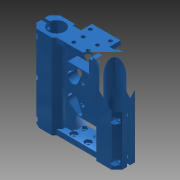
# Autodesk Inventor part: ChimeraXCarriage4
Saved by Autodesk Inventor 2015 SP1 (Build 190203100, 203)
## iProperties
Created: 2015-01-02
Part Number: ChimeraXCarriage4
Material: ABS Plastic
Document SubType Name: Modeling
Designer: Jack
Density: 1.06 g/cm^3
Appearance: Cyan
Mass: 64.3175 g
Surface Area: 300.836 cm^2
Volume: 60.6769 cm^3
Author: Jack
Autodesk Inventor part; units mm, degrees
ref_plane "YZ Plane" through (0, 0, 0) normal (1, 0, 0) x (0, 1, 0)
ref_plane "XZ Plane" through (0, 0, 0) normal (0, 1, 0) x (-1, 0, 0)
ref_plane "XY Plane" through (0, 0, 0) normal (0, 0, 1) x (1, 0, 0)
sketch "Sketch1" plane through (0, 0, 0) normal (0, 0, 1) x (1, 0, 0)
  arc A0 (-7.6035, -1.5) -> (-7.6035, 1.5) centre (0, 0) ccw
  arc A1 (62.6035, 1.5) -> (62.6035, -1.5) centre (55, 0) ccw
  line L0 (-7.6035, 1.5) -> (-13, 1.5)
  line L1 (-13, 1.5) -> (-13, 11)
  line L2 (-13, 11) -> (11.5, 11)
  line L3 (11.5, 11) -> (11.5, 6)
  line L4 (11.5, 6) -> (43.5, 6)
  line L5 (43.5, 6) -> (43.5, 11)
  line L6 (43.5, 11) -> (68, 11)
  line L7 (68, 11) -> (68, 1.5)
  line L8 (68, 1.5) -> (62.6035, 1.5)
  line L9 (62.6035, -1.5) -> (68, -1.5)
  line L10 (68, -1.5) -> (68, -11)
  line L11 (-13, -11) -> (-13, -1.5)
  line L12 (-13, -1.5) -> (-7.6035, -1.5)
  line L13 (-13, -11) -> (11.5, -11)
  line L14 (11.5, -11) -> (11.5, -3)
  line L15 (11.5, -3) -> (43.5, -3)
  line L16 (43.5, -3) -> (43.5, -11)
  line L17 (43.5, -11) -> (68, -11)
  dimension "d0" = 15.5
  dimension "d1" = 15.5
  dimension "d2" = 55
  dimension "d3" = 1.5
  dimension "d4" = 13
  dimension "d5" = 11
  dimension "d6" = 11
  dimension "d7" = 11.5
  dimension "d8" = 11.5
  dimension "d9" = 5
  dimension "d10" = 8
  constraints: 36 end point, 11 perpendicular, 7 point on line, 4 horizontal alignment, 4 point on circle, 3 equal length, 3 horizontal, 2 centre point, 2 vertical alignment, 1 coincident, 1 parallel
  measures "d0" diameter of A0
  measures "d1" diameter of A1
  measures "d2" distance of point (0, 0) A1.centre
  measures "d3" distance from line of point (0, 0) L0
  measures "d4" distance from line of point (0, 0) L1
  measures "d5" distance from line of L2 point (0, 0)
  measures "d6" distance from line of L13 point (0, 0)
  measures "d7" distance from line of L3 point (0, 0)
  measures "d8" distance from line of L5 A1.centre
  measures "d9" distance of L2.end L3.end
  measures "d10" distance of L13.end L14.end
extrude "Extrusion1" add sketch "Sketch1" along normal blind 80
chamfer "Chamfer1" distance 5 angle 45 4 edges at (-13, 11, 40) (-13, -11, 40) (68, 11, 40) (68, -11, 40)
chamfer "Chamfer2" distance 5 angle 45 2 edges at (11.5, 11, 40) (43.5, 11, 40)
chamfer "Chamfer3" distance 5 angle 45 2 edges at (11.5, -11, 40) (43.5, -11, 40)
sketch "Sketch2" plane through (0, 0, 80) normal (0, 0, 1) x (1, 0, 0)
  line L0 (48.5, -11) -> (43.5, -6) projected
  line L1 (48.5, -11) -> (63, -11) projected
  line L2 (63, 11) -> (48.5, 11) projected
  line L3 (43.5, 6) -> (48.5, 11) projected
  line L4 (43.5, 6) -> (11.5, 6) projected
  line L5 (6.5, 11) -> (11.5, 6) projected
  line L6 (11.5, -6) -> (11.5, -3) projected
  line L7 (11.5, -3) -> (43.5, -3) projected
  line L8 (43.5, -3) -> (43.5, -6) projected
  line L9 (8.8, 8.7) -> (46.2, 8.7)
  line L10 (6.5, -11) -> (11.5, -6) projected
  line L11 (8.8, -8.7) -> (46.2, -8.7)
  dimension "d22" = 2.3
  dimension "d23" = 2.3
  constraints: 4 end point, 4 point on line, 1 horizontal, 1 parallel
  measures "d22" distance between parallel lines of L1 L11
  measures "d23" distance between parallel lines of L2 L9
extrude "Extrusion2" add sketch "Sketch2" against normal blind 5
sketch "Sketch3" plane through (0, 0, 0) normal (0, 0, -1) x (-1, 0, 0)
  line L0 (-43.5, -6) -> (-48.5, -11) projected
  line L1 (-43.5, -3) -> (-43.5, -6) projected
  line L2 (-11.5, -3) -> (-43.5, -3) projected
  line L3 (-11.5, -6) -> (-11.5, -3) projected
  line L4 (-6.5, -11) -> (-11.5, -6) projected
  line L5 (-11.5, 6) -> (-6.5, 11) projected
  line L6 (-43.5, 6) -> (-11.5, 6) projected
  line L7 (-48.5, 11) -> (-43.5, 6) projected
  line L8 (-8.8, 8.7) -> (-46.2, 8.7) projected
  line L9 (-46.2, -8.7) -> (-8.8, -8.7) projected
extrude "Extrusion3" add sketch "Sketch3" against normal blind 5
sketch "Sketch4" plane through (11.5, 6, 75) normal (0, 1, 0) x (1, 0, 0)
  line L0 (0, 0) -> (32, 0) projected
  line L1 (0, 70) -> (32, 70) projected
  line L2 (30, 70) -> (10, 70)
  line L3 (10, 70) -> (10, 55)
  line L4 (10, 55) -> (30, 55)
  line L5 (30, 55) -> (30, 70)
  line L6 (22, 0) -> (2, 0)
  line L7 (2, 0) -> (2, 15)
  line L8 (2, 15) -> (22, 15)
  line L9 (22, 15) -> (22, 0)
  line L10 (0, 70) -> (0, 0) projected
  line L11 (32, 70) -> (32, 0) projected
  point P0 (-11.5, 75)
  dimension "d28" = 20
  dimension "d29" = 15
  dimension "d33" = 2
  dimension "d34" = 2
  constraints: 16 end point, 6 parallel, 2 horizontal, 2 perpendicular, 2 point on line
  measures "d28" distance of L4.end L3.end
  measures "d29" distance of L3.end L2.end
  measures "d33" distance between parallel lines of L10 L7
  measures "d34" distance between parallel lines of L11 L5
extrude "Extrusion4" cut sketch "Sketch4" against normal up to next contours L7 L8 L9 L0 | L1 L5 L4 L3
sketch "Sketch5" plane through (43.5, 6, 75) normal (0, 1, 0) x (1, 0, 0)
  line L0 (-10, 0) -> (0, 0) projected
  line L1 (0, 70) -> (0, 0) projected
  circle A0 centre (-16, 44) radius 1.75
  circle A1 centre (-16, 26) radius 1.75
  point P0 (-43.5, 75)
  dimension "d35" = 3.5
  dimension "d36" = 3.5
  dimension "d37" = 16
  dimension "d38" = 18
  dimension "d39" = 26
  constraints: 2 centre point, 1 vertical alignment
  measures "d35" diameter of A0
  measures "d36" diameter of A1
  measures "d37" distance from line of L1 A1.centre
  measures "d38" distance of A0.centre A1.centre
  measures "d39" distance from line of L0 A1.centre
extrude "Extrusion5" cut sketch "Sketch5" against normal up to next
sketch "Sketch6" plane through (43.5, 6, 75) normal (0, 1, 0) x (1, 0, 0)
  circle A0 centre (-16, 44) radius 1.75 projected
  circle A1 centre (-16, 26) radius 1.75 projected
  circle A2 centre (-25, 44) radius 5
  circle A3 centre (-25, 26) radius 5
  point P0 (-43.5, 75)
  dimension "d42" = 10
  dimension "d43" = 9
  constraints: 2 centre point, 2 horizontal alignment, 1 equal radius, 1 vertical alignment
  measures "d42" diameter of A2
  measures "d43" distance of A1.centre A3.centre
extrude "Extrusion6" cut sketch "Sketch6" against normal up to next contours A2 | A3
sketch "Sketch7" plane through (43.5, 6, 75) normal (0, 1, 0) x (1, 0, 0)
  circle A0 centre (-25, 44) radius 5 projected
  circle A1 centre (-25, 26) radius 5 projected
  arc A2 (-20.5127, 16.3096) -> (-16.7002, 19.2803) centre (-19, 18.3) ccw
  arc A3 (-16.7002, 50.7197) -> (-20.5127, 53.6904) centre (-19, 51.7) ccw
  line L0 (-16.7002, 50.7197) -> (-20.4005, 42.0393)
  line L1 (-20.5127, 53.6904) -> (-28.0254, 47.9808)
  line L2 (-16.7002, 19.2803) -> (-20.4005, 27.9607)
  line L3 (-20.5127, 16.3096) -> (-28.0254, 22.0192)
  point P0 (-43.5, 75)
  dimension "d46" = 7.7
  dimension "d47" = 7.7
  dimension "d48" = 6
  dimension "d49" = 5
  dimension "d50" = 6
  constraints: 8 end point, 8 point on circle, 8 tangent, 2 centre point, 1 equal radius
  measures "d46" vertical distance of A0.centre A3.centre
  measures "d47" vertical distance of A2.centre A1.centre
  measures "d48" horizontal distance of A1.centre A2.centre
  measures "d49" diameter of A3
  measures "d50" horizontal distance of A0.centre A3.centre
extrude "Extrusion7" cut sketch "Sketch7" against normal up to next contours A0 L1 A3 L0 | A1 L2 A2 L3
sketch "Sketch8" plane through (0, 0, 0) normal (0, 0, -1) x (-1, 0, 0)
  arc A0 (7.6035, 1.5) -> (7.6035, -1.5) centre (0, 0) ccw projected
  line L0 (-8.8, 8.7) -> (-46.2, 8.7) projected
  circle A1 centre (-34.25, 4.45) radius 1.75
  circle A2 centre (-20.75, 4.45) radius 1.75
  circle A3 centre (-34.25, -4.45) radius 1.75
  circle A4 centre (-20.75, -4.45) radius 1.75
  dimension "d53" = 13.5
  dimension "d54" = 8.9
  dimension "d55" = 3.5
  dimension "d56" = 4.25
  dimension "d57" = 20.75
  constraints: 4 centre point, 3 equal radius, 2 horizontal alignment, 2 vertical alignment
  measures "d53" distance of A4.centre A3.centre
  measures "d54" distance of A4.centre A2.centre
  measures "d55" diameter of A2
  measures "d56" distance from line of L0 A2.centre
  measures "d57" horizontal distance of A0.centre A4.centre
extrude "Extrusion8" cut sketch "Sketch8" against normal up to surface (5 mm away)
sketch "Sketch9" plane through (0, 0, 75) normal (0, 0, -1) x (-1, 0, 0)
  circle A0 centre (-34.25, 4.45) radius 1.75 projected
  circle A1 centre (-34.25, -4.45) radius 1.75 projected
  circle A2 centre (-20.75, -4.45) radius 1.75 projected
  circle A3 centre (-20.75, 4.45) radius 1.75 projected
  point P0 (0, 0)
extrude "Extrusion9" cut sketch "Sketch9" against normal up to next
sketch "Sketch12" plane through (0, 0, 75) normal (0, 0, -1) x (-1, 0, 0)
  arc A0 (-35.2298, -3) -> (-33.5, -2.8689) centre (-34.25, -4.45) ccw projected
  arc A1 (-33.5, 2.8689) -> (-35.0624, 6) centre (-34.25, 4.45) ccw projected
  circle A2 centre (-20.75, -4.45) radius 1.75 projected
  circle A3 centre (-20.75, 4.45) radius 1.75 projected
  line L0 (-34.25, -1.0436) -> (-31.3, -2.7468)
  line L1 (-31.3, -2.7468) -> (-31.3, -6.1532)
  line L2 (-31.3, -6.1532) -> (-34.25, -7.8564)
  line L3 (-34.25, -7.8564) -> (-37.2, -6.1532)
  line L4 (-37.2, -6.1532) -> (-37.2, -2.7468)
  line L5 (-37.2, -2.7468) -> (-34.25, -1.0436)
  line L6 (-20.75, -1.0436) -> (-17.8, -2.7468)
  line L7 (-17.8, -2.7468) -> (-17.8, -6.1532)
  line L8 (-17.8, -6.1532) -> (-20.75, -7.8564)
  line L9 (-20.75, -7.8564) -> (-23.7, -6.1532)
  line L10 (-23.7, -6.1532) -> (-23.7, -2.7468)
  line L11 (-23.7, -2.7468) -> (-20.75, -1.0436)
  line L12 (-20.75, 7.8564) -> (-17.8, 6.1532)
  line L13 (-17.8, 6.1532) -> (-17.8, 2.7468)
  line L14 (-17.8, 2.7468) -> (-20.75, 1.0436)
  line L15 (-20.75, 1.0436) -> (-23.7, 2.7468)
  line L16 (-23.7, 2.7468) -> (-23.7, 6.1532)
  line L17 (-23.7, 6.1532) -> (-20.75, 7.8564)
  line L18 (-34.25, 7.8564) -> (-31.3, 6.1532)
  line L19 (-31.3, 6.1532) -> (-31.3, 2.7468)
  line L20 (-31.3, 2.7468) -> (-34.25, 1.0436)
  line L21 (-34.25, 1.0436) -> (-37.2, 2.7468)
  line L22 (-37.2, 2.7468) -> (-37.2, 6.1532)
  line L23 (-37.2, 6.1532) -> (-34.25, 7.8564)
  point P0 (0, 0)
  dimension "d80" = 5.9
  constraints: 48 end point, 4 coincident, 4 vertical, 3 equal length, 52 other
  measures "d80" distance between parallel lines of L4 L1
extrude "Extrusion14" cut sketch "Sketch12" along normal blind 2.7 and the other way blind 2.7 contours A2 | A3 | L0 L1 L2 L3 L4 L5 | L6 L7 L8 L9 L10 L11 | L12 L13 L14 L15 L16 L17 | L18 L19 L20 L21 L22 L23
sketch "Sketch13" plane through (0, 0, 5) normal (0, 0, 1) x (1, 0, 0)
  circle A0 centre (34.25, 4.45) radius 1.75 projected
  circle A1 centre (34.25, -4.45) radius 1.75 projected
  circle A2 centre (34.25, 4.45) radius 1.75 projected
  line L0 (34.25, 7.8564) -> (31.3, 6.1532) projected
  line L1 (37.2, 6.1532) -> (34.25, 7.8564) projected
  line L2 (37.2, 2.7468) -> (37.2, 6.1532) projected
  line L3 (34.25, 1.0436) -> (37.2, 2.7468) projected
  line L4 (31.3, 2.7468) -> (34.25, 1.0436) projected
  line L5 (31.3, 6.1532) -> (31.3, 2.7468) projected
  circle A3 centre (20.75, 4.45) radius 1.75 projected
  line L6 (20.75, 7.8564) -> (17.8, 6.1532) projected
  line L7 (23.7, 6.1532) -> (20.75, 7.8564) projected
  line L8 (23.7, 2.7468) -> (23.7, 6.1532) projected
  line L9 (20.75, 1.0436) -> (23.7, 2.7468) projected
  line L10 (17.8, 2.7468) -> (20.75, 1.0436) projected
  line L11 (17.8, 6.1532) -> (17.8, 2.7468) projected
  circle A4 centre (20.75, -4.45) radius 1.75 projected
  line L12 (20.75, -1.0436) -> (17.8, -2.7468) projected
  line L13 (23.7, -2.7468) -> (20.75, -1.0436) projected
  line L14 (23.7, -6.1532) -> (23.7, -2.7468) projected
  line L15 (20.75, -7.8564) -> (23.7, -6.1532) projected
  line L16 (17.8, -6.1532) -> (20.75, -7.8564) projected
  line L17 (17.8, -2.7468) -> (17.8, -6.1532) projected
  circle A5 centre (34.25, -4.45) radius 1.75 projected
  line L18 (34.25, -1.0436) -> (31.3, -2.7468) projected
  line L19 (37.2, -2.7468) -> (34.25, -1.0436) projected
  line L20 (37.2, -6.1532) -> (37.2, -2.7468) projected
  line L21 (34.25, -7.8564) -> (37.2, -6.1532) projected
  line L22 (31.3, -6.1532) -> (34.25, -7.8564) projected
  line L23 (31.3, -2.7468) -> (31.3, -6.1532) projected
  point P0 (0, 0)
extrude "Extrusion15" cut sketch "Sketch13" along normal blind 2.7 and the other way blind 2.7 contours A0 | A1 | L1 L2 L3 L4 L5 L0 | A3 | L7 L8 L9 L10 L11 L6 | A4 | L13 L14 L15 L16 L17 L12 | L19 L20 L21 L22 L23 L18
sketch "Sketch14" plane through (0, 0, 5) normal (0, 0, 1) x (1, 0, 0)
  line L0 (23.7, 2.7468) -> (21.5, 1.4766) projected
  line L1 (21.5, 1.4766) -> (21.5, -1.4766) projected
  line L2 (21.5, -1.4766) -> (23.7, -2.7468) projected
  line L3 (23.7, -2.7468) -> (23.7, -6.1532) projected
  line L4 (23.7, -6.1532) -> (20.75, -7.8564) projected
  line L5 (20.75, -7.8564) -> (17.8, -6.1532) projected
  line L6 (17.8, -6.1532) -> (17.8, -3) projected
  line L7 (17.8, 6) -> (17.8, 6.1532) projected
  line L8 (17.8, 6.1532) -> (20.75, 7.8564) projected
  line L9 (20.75, 7.8564) -> (23.7, 6.1532) projected
  line L10 (23.7, 6.1532) -> (23.7, 2.7468) projected
  line L11 (17.8, 6) -> (17.8, -3)
  point P0 (0, 0)
  constraints: 2 end point, 1 collinear
extrude "Extrusion16" cut sketch "Sketch14" along normal blind 2.7
sketch "Sketch15" plane through (0, 0, 75) normal (0, 0, -1) x (-1, 0, 0)
  line L0 (-31.3, 2.7468) -> (-33.5, 1.4766) projected
  line L1 (-33.5, 1.4766) -> (-33.5, -1.4766) projected
  line L2 (-33.5, -1.4766) -> (-31.3, -2.7468) projected
  line L3 (-31.3, -2.7468) -> (-31.3, -6.1532) projected
  line L4 (-31.3, -6.1532) -> (-34.25, -7.8564) projected
  line L5 (-34.25, -7.8564) -> (-37.2, -6.1532) projected
  line L6 (-37.2, -6.1532) -> (-37.2, -3) projected
  line L7 (-37.2, 6.1532) -> (-34.25, 7.8564) projected
  line L8 (-34.25, 7.8564) -> (-31.3, 6.1532) projected
  line L9 (-31.3, 6.1532) -> (-31.3, 2.7468) projected
  line L10 (-37.2, 6) -> (-37.2, -3)
  line L11 (-37.2, 2.7468) -> (-37.2, 6.1532) projected
  point P0 (0, 0)
  constraints: 2 end point, 1 collinear
extrude "Extrusion17" cut sketch "Sketch15" along normal blind 2.7
sketch "Sketch16" plane through (63, 11, 80) normal (0, 1, 0) x (1, 0, 0)
  line L0 (0, 0) -> (-14.5, 0) projected
  line L1 (0, 80) -> (0, 0) projected
  line L2 (0, 80) -> (-14.5, 80) projected
  line L3 (-56.5, 80) -> (-56.5, 0) projected
  line L4 (-56.5, 80) -> (-71, 80) projected
  line L5 (-71, 0) -> (-71, 80) projected
  line L6 (-56.5, 0) -> (-71, 0) projected
  circle A0 centre (1.5, 6) radius 1.75
  circle A1 centre (1.5, 74) radius 1.75
  circle A2 centre (1.5, 40) radius 1.75
  circle A3 centre (-72.5, 6) radius 1.75
  circle A4 centre (-72.5, 40) radius 1.75
  circle A5 centre (-72.5, 74) radius 1.75
  line L7 (5, 80) -> (0, 80) projected
  point P0 (-63, 80)
  dimension "d93" = 3.5
  dimension "d94" = 1.5
  dimension "d95" = 1.5
  dimension "d96" = 6
  dimension "d97" = 6
  dimension "d107" = 40
  constraints: 6 centre point, 5 equal radius, 4 vertical alignment, 3 horizontal alignment
  measures "d93" diameter of A0
  measures "d94" distance from line of L5 A3.centre
  measures "d95" distance from line of L1 A0.centre
  measures "d96" distance from line of L0 A0.centre
  measures "d97" distance from line of L2 A1.centre
  measures "d107" distance from line of L7 A2.centre
extrude "Extrusion18" cut sketch "Sketch16" against normal up to surface contours A1 L1 | L1 A1 | A2 L1 | L1 A2 | A0 L1 | L1 A0 | A5 L5 | L5 A5 | A3 L5 | L5 A3 | A4 L5 | L5 A4 surface through (65.5, -8.5, 0) normal (0.7071068, -0.7071068, 0)
sketch "Sketch17" plane through (-8, 11, 80) normal (0, 1, 0) x (1, 0, 0)
  line L0 (56.5, 0) -> (56.5, 80) projected
  line L1 (71, 0) -> (56.5, 0) projected
  line L2 (71, 80) -> (71, 74.9014) projected
  line L3 (71, 80) -> (56.5, 80) projected
  circle A0 centre (72.5, 6) radius 1.75 projected
  circle A1 centre (72.5, 40) radius 1.75 projected
  circle A2 centre (72.5, 74) radius 1.75 projected
  circle A3 centre (-1.5, 74) radius 1.75 projected
  circle A4 centre (-1.5, 40) radius 1.75 projected
  circle A5 centre (-1.5, 6) radius 1.75 projected
  circle A6 centre (-1.5, 6) radius 3.65
  circle A7 centre (-1.5, 40) radius 3.65
  circle A8 centre (-1.5, 74) radius 3.65
  circle A9 centre (72.5, 74) radius 3.65
  circle A10 centre (72.5, 40) radius 3.65
  circle A11 centre (72.5, 6) radius 3.65
  arc A12 (71, 74.9014) -> (71, 73.0986) centre (72.5, 74) ccw projected
  line L4 (71, 5.0986) -> (71, 0) projected
  arc A13 (71, 6.9014) -> (71, 5.0986) centre (72.5, 6) ccw projected
  line L5 (71, 39.0986) -> (71, 6.9014) projected
  arc A14 (71, 40.9014) -> (71, 39.0986) centre (72.5, 40) ccw projected
  line L6 (71, 73.0986) -> (71, 40.9014) projected
  point P0 (8, 80)
  dimension "d101" = 7.3
  constraints: 6 centre point, 6 coincident, 5 equal radius
  measures "d101" diameter of A6
extrude "Extrusion19" cut sketch "Sketch17" against normal blind 5 contours L4 A0 L5 A11 | A11 L5 A0 L4 | A9 L6 A2 L2 | L2 A2 L6 A9 | A0 | A2 | L5 A1 L6 A10 | A10 L6 A1 L5 | A1 | A3 | A4 | A5 | A6 | A7 | A8
sketch "Sketch18" plane through (-8, -11, 0) normal (0, -1, 0) x (1, 0, 0)
  line L0 (56.5, 0) -> (56.5, 80)
  line L1 (56.5, 0) -> (71, 0)
  line L2 (71, 80) -> (71, 74.9014)
  line L3 (56.5, 80) -> (71, 80)
  circle A0 centre (-1.5, 74) radius 1.75
  arc A1 (0, 74.9014) -> (0, 73.0986) centre (-1.5, 74) ccw
  circle A2 centre (-1.5, 40) radius 1.75
  arc A3 (0, 40.9014) -> (0, 39.0986) centre (-1.5, 40) ccw
  circle A4 centre (-1.5, 6) radius 1.75
  arc A5 (0, 6.9014) -> (0, 5.0986) centre (-1.5, 6) ccw
  arc A6 (71, 5.0986) -> (71, 6.9014) centre (72.5, 6) ccw
  circle A7 centre (72.5, 6) radius 1.75
  arc A8 (71, 39.0986) -> (71, 40.9014) centre (72.5, 40) ccw
  circle A9 centre (72.5, 40) radius 1.75
  arc A10 (71, 73.0986) -> (71, 74.9014) centre (72.5, 74) ccw
  circle A11 centre (72.5, 74) radius 1.75
  line L4 (-1.5, 77.1754) -> (1.25, 75.5877)
  line L5 (1.25, 75.5877) -> (1.25, 72.4123)
  line L6 (1.25, 72.4123) -> (-1.5, 70.8246)
  line L7 (-1.5, 70.8246) -> (-4.25, 72.4123)
  line L8 (-4.25, 72.4123) -> (-4.25, 75.5877)
  line L9 (-4.25, 75.5877) -> (-1.5, 77.1754)
  line L10 (-4.25, 41.5877) -> (-1.5, 43.1754)
  line L11 (-1.5, 43.1754) -> (1.25, 41.5877)
  line L12 (1.25, 41.5877) -> (1.25, 38.4123)
  line L13 (1.25, 38.4123) -> (-1.5, 36.8246)
  line L14 (-1.5, 36.8246) -> (-4.25, 38.4123)
  line L15 (-4.25, 38.4123) -> (-4.25, 41.5877)
  circle A12 centre (-1.5, 6) radius 1.75
  line L16 (-4.25, 7.5877) -> (-1.5, 9.1754)
  line L17 (-1.5, 9.1754) -> (1.25, 7.5877)
  line L18 (1.25, 7.5877) -> (1.25, 4.4123)
  line L19 (1.25, 4.4123) -> (-1.5, 2.8246)
  line L20 (-1.5, 2.8246) -> (-4.25, 4.4123)
  line L21 (-4.25, 4.4123) -> (-4.25, 7.5877)
  line L22 (72.5, 77.1754) -> (75.25, 75.5877)
  line L23 (75.25, 75.5877) -> (75.25, 72.4123)
  line L24 (75.25, 72.4123) -> (72.5, 70.8246)
  line L25 (72.5, 70.8246) -> (69.75, 72.4123)
  line L26 (69.75, 72.4123) -> (69.75, 75.5877)
  line L27 (69.75, 75.5877) -> (72.5, 77.1754)
  line L28 (75.25, 41.5877) -> (75.25, 38.4123)
  line L29 (75.25, 38.4123) -> (72.5, 36.8246)
  line L30 (72.5, 36.8246) -> (69.75, 38.4123)
  line L31 (69.75, 38.4123) -> (69.75, 41.5877)
  line L32 (69.75, 41.5877) -> (72.5, 43.1754)
  line L33 (72.5, 43.1754) -> (75.25, 41.5877)
  line L34 (75.25, 7.5877) -> (75.25, 4.4123)
  line L35 (75.25, 4.4123) -> (72.5, 2.8246)
  line L36 (72.5, 2.8246) -> (69.75, 4.4123)
  line L37 (69.75, 4.4123) -> (69.75, 7.5877)
  line L38 (69.75, 7.5877) -> (72.5, 9.1754)
  line L39 (72.5, 9.1754) -> (75.25, 7.5877)
  arc A13 (71, 74.9014) -> (71, 73.0986) centre (72.5, 74) ccw
  arc A14 (71, 40.9014) -> (71, 39.0986) centre (72.5, 40) ccw
  arc A15 (71, 6.9014) -> (71, 5.0986) centre (72.5, 6) ccw
  arc A16 (0, 5.0986) -> (0, 6.9014) centre (-1.5, 6) ccw
  arc A17 (0, 39.0986) -> (0, 40.9014) centre (-1.5, 40) ccw
  arc A18 (0, 73.0986) -> (0, 74.9014) centre (-1.5, 74) ccw
  arc A19 (71, 6.9014) -> (71, 5.0986) centre (72.5, 6) ccw
  line L40 (71, 39.0986) -> (71, 6.9014)
  arc A20 (71, 40.9014) -> (71, 39.0986) centre (72.5, 40) ccw
  line L41 (71, 73.0986) -> (71, 40.9014)
  arc A21 (71, 74.9014) -> (71, 73.0986) centre (72.5, 74) ccw
  line L42 (71, 5.0986) -> (71, 0)
  point P0 (8, 0)
  point P1 (-1.5, 74)
  point P2 (-1.5, 40)
  point P3 (-1.5, 6)
extrude "Extrusion20" cut sketch "Sketch18" against normal blind 5 contours L42 A6 L40 L38 L39 L34 L35 L36 | L36 L37 L38 L40 A7 L42 | L27 L22 L23 L24 L25 L41 A10 L2 | L2 A11 L41 L25 L26 L27 | L40 A8 L41 L32 L33 L28 L29 L30 | L30 L31 L32 L41 A9 L40 | L4 L5 L6 L7 L8 L9 | L10 L11 L12 L13 L14 L15 | L16 L17 L18 L19 L20 L21
sketch "Sketch19" plane through (0, 0, 80) normal (0, 0, 1) x (1, 0, 0)
  line L0 (46.2, 8.7) -> (8.8, 8.7) projected
  line L1 (14.3, 19.2) -> (41.3, 19.2)
  line L2 (41.3, 19.2) -> (41.3, 8.7)
  line L3 (46.2, 8.7) -> (8.8, 8.7) projected
  line L4 (14.3, 19.2) -> (14.3, 8.7)
  dimension "d109" = 27
  dimension "d110" = 5.5
  dimension "d111" = 10.5
  constraints: 6 end point, 2 perpendicular, 2 point on line, 1 horizontal
  measures "d109" distance of L1.start L1.end
  measures "d110" distance from line of L0.end L4
  measures "d111" distance between parallel lines of L0 L1
extrude "Extrusion21" add sketch "Sketch19" against normal blind 4
sketch "Sketch20" plane through (0, 0, 80) normal (0, 0, 1) x (1, 0, 0)
  line L0 (41.3, 19.2) -> (14.3, 19.2) projected
  circle A0 centre (18, 13.95) radius 1.75
  circle A1 centre (37, 13.95) radius 1.75
  line L1 (14.3, 19.2) -> (14.3, 8.7) projected
  dimension "d114" = 5.25
  dimension "d115" = 3.5
  dimension "d117" = 19
  dimension "d120" = 3.7
  constraints: 2 centre point, 1 equal radius, 1 horizontal alignment
  measures "d114" distance from line of L0 A1.centre
  measures "d115" diameter of A1
  measures "d117" distance of A1.centre A0.centre
  measures "d120" distance from line of L1 A0.centre
extrude "Extrusion22" cut sketch "Sketch20" against normal up to next
sketch "Sketch21" plane through (0, 0, 76) normal (0, 0, -1) x (-1, 0, 0)
  circle A0 centre (-18, 13.95) radius 1.75 projected
  circle A1 centre (-37, 13.95) radius 1.75 projected
  line L0 (-37, 17.2986) -> (-34.1, 15.6243)
  line L1 (-34.1, 15.6243) -> (-34.1, 12.2757)
  line L2 (-34.1, 12.2757) -> (-37, 10.6014)
  line L3 (-37, 10.6014) -> (-39.9, 12.2757)
  line L4 (-39.9, 12.2757) -> (-39.9, 15.6243)
  line L5 (-39.9, 15.6243) -> (-37, 17.2986)
  line L6 (-18, 17.2986) -> (-15.1, 15.6243)
  line L7 (-15.1, 15.6243) -> (-15.1, 12.2757)
  line L8 (-15.1, 12.2757) -> (-18, 10.6014)
  line L9 (-18, 10.6014) -> (-20.9, 12.2757)
  line L10 (-20.9, 12.2757) -> (-20.9, 15.6243)
  line L11 (-20.9, 15.6243) -> (-18, 17.2986)
  point P0 (0, 0)
  dimension "d121" = 5.8
  constraints: 24 end point, 2 coincident, 2 vertical, 1 parallel, 26 other
  measures "d121" distance between parallel lines of L1 L4
extrude "Extrusion23" cut sketch "Sketch21" against normal blind 2.6
sketch "Sketch22" plane through (0, 0, 80) normal (0, 0, 1) x (1, 0, 0)
  line L0 (6.5, 11) -> (8.8, 8.7) projected
  line L1 (6.5, 11) -> (6.5, 8.7)
  line L2 (6.5, 8.7) -> (8.8, 8.7)
  constraints: 4 end point, 1 perpendicular, 1 vertical
extrude "Extrusion24" cut sketch "Sketch22" against normal blind 8
body "Solid1"
